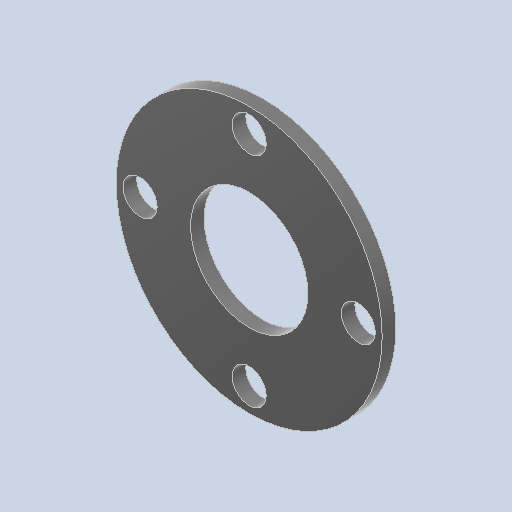
# Autodesk Inventor part: rotor_shim
Saved by Autodesk Inventor 2024.3 (Build 283343010, 343A)
## iProperties
Created: 2025-06-29
Part Number: rotor_shim
Material: 一般
Document SubType Name: Modeling
Designer: kshau
Density: 1 g/cm^3
Appearance: 滑らか - 黒
Author: kshau
Autodesk Inventor part; units mm, degrees
ref_plane "YZ Plane" through (0, 0, 0) normal (1, 0, 0) x (0, 1, 0)
ref_plane "XZ Plane" through (0, 0, 0) normal (0, 1, 0) x (-1, 0, 0)
ref_plane "XY Plane" through (0, 0, 0) normal (0, 0, 1) x (1, 0, 0)
sketch "スケッチ1" plane through (0, 0, 0) normal (0, 0, 1) x (1, 0, 0)
  circle A0 centre (0, 0) radius 9.75
  circle A1 centre (0, 0) radius 4.3
  dimension "d0" = 19.5
  dimension "d1" = 8.6
  constraints: 2 centre point, 2 coincident
  measures "d0" diameter of A0
  measures "d1" diameter of A1
extrude "押し出し1" add sketch "スケッチ1" along normal blind 1
sketch "スケッチ2" plane through (0, 0, 1) normal (0, 0, 1) x (1, 0, 0)
  circle A0 centre (0, 0) radius 8
  point P0 (0, 8)
  point P1 (-8, 0)
  point P2 (0, -8)
  point P3 (8, 0)
  dimension "d4" = 16
  dimension "d7" = 360
  constraints: 1 coincident, 1 vertical alignment, 7 other
hole "穴1" at (0, 8, 1) at (-8, 0, 1) at (0, -8, 1) at (8, 0, 1) direction (0, 0, -1) diameter 2.5 end through all
